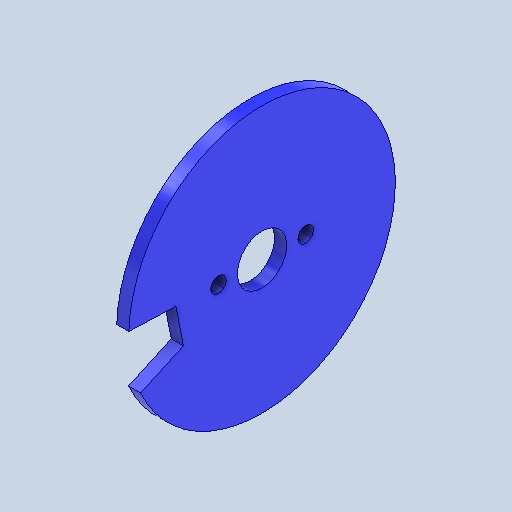
# Autodesk Inventor part: belt_liner_v3_3DP_P-2-F
Saved by Autodesk Inventor 2025.2 (Build 292293000, 293)
## iProperties
Created: 2025-01-19
Part Number: belt_liner_v3_3DP_P-2-F
Material: ABS プラスチック
Document SubType Name: Modeling
Designer: haruy
Density: 1.06 g/cm^3
Appearance: 青 - 壁塗料 - 光沢
Author: haruy
Autodesk Inventor part; units mm, degrees
ref_plane "YZ Plane" through (0, 0, 0) normal (1, 0, 0) x (0, 1, 0)
ref_plane "XZ Plane" through (0, 0, 0) normal (0, 1, 0) x (-1, 0, 0)
ref_plane "XY Plane" through (0, 0, 0) normal (0, 0, 1) x (1, 0, 0)
sketch "スケッチ1" plane through (0, 0, 0) normal (1, 0, 0) x (0, 1, 0)
  line L0 (-2.4757, 20.6884) -> (-6.5003, 29.5193)
  arc A0 (-6.5003, 29.5193) -> (5.7094, 31.948) centre (4.8303, 4.4621) ccw
  line L1 (5.7094, 31.948) -> (5.3706, 22.2491)
  line L2 (5.3706, 22.2491) -> (-2.4757, 20.6884)
  circle A1 centre (4.8303, -4.5379) radius 1.6
  circle A2 centre (4.8303, 13.4621) radius 1.6
  circle A3 centre (4.8303, 4.4621) radius 5.1
  point P0 (0, 0)
  constraints: 6 end point, 4 centre point, 2 point on circle
extrude "押し出し1" add sketch "スケッチ1" against normal blind 2.5
